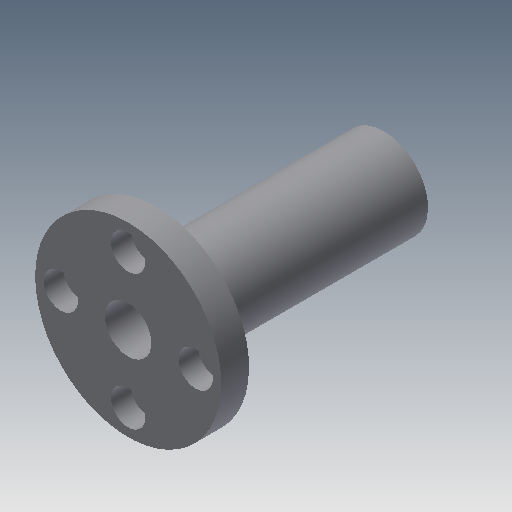
# Autodesk Inventor part: NB_SMF10WW
Saved by Autodesk Inventor 2019.4 (Build 234330000, 330)
## iProperties
Created: 2018-08-09
Part Number: NB_SMF10WW
Material: 一般
Document SubType Name: Modeling
Designer: Owner
Density: 1 g/cm^3
Appearance: 既定
Mass: 16.2699 g
Surface Area: 81.3509 cm^2
Volume: 16.2699 cm^3
Author: Owner
Autodesk Inventor part; units mm, degrees
ref_plane "YZ Plane" through (0, 0, 0) normal (1, 0, 0) x (0, 1, 0)
ref_plane "XZ Plane" through (0, 0, 0) normal (0, 1, 0) x (-1, 0, 0)
ref_plane "XY Plane" through (0, 0, 0) normal (0, 0, 1) x (1, 0, 0)
sketch "スケッチ2" plane through (0, 0, 0) normal (1, 0, 0) x (0, 1, 0)
  line L0 (5, 0) -> (9.5, 0)
  line L1 (9.5, 0) -> (9.5, 49)
  line L2 (9.5, 49) -> (20, 49)
  line L3 (20, 49) -> (20, 55)
  line L4 (20, 55) -> (5, 55)
  line L5 (5, 0) -> (5, 55)
  line L6 (0, -11) -> (0, 66) projected
  point P0 (0, 0)
  point P1 (0, 55)
  dimension "d0" = 9.5
  dimension "d1" = 55
  dimension "d2" = 6
  dimension "d3" = 20
  dimension "d4" = 5
  constraints: 12 end point, 4 perpendicular, 2 point on line, 1 horizontal, 1 vertical, 1 vertical alignment
  measures "d0" distance of point (0, 0) L0.end
  measures "d1" distance between parallel lines of L4 L0
  measures "d2" distance of L2.end L3.end
  measures "d3" distance of L3.end point (0, 55)
  measures "d4" distance from line of point (0, 0) L5
revolve "回転1" add sketch "スケッチ2" angle 360 about axis through (0, 0, -10) along (0, 0, 1)
sketch "スケッチ3" plane through (0, 0, 55) normal (0, 0, 1) x (1, 0, 0)
  circle A0 centre (0, 14.5) radius 3.7
  point P0 (0, 0)
  dimension "d6" = 14.5
  dimension "d7" = 7.4
  constraints: 1 centre point, 1 vertical alignment
  measures "d6" distance of point (0, 0) A0.centre
  measures "d7" diameter of A0
extrude "押し出し1" cut sketch "スケッチ3" against normal blind 4.3
sketch "スケッチ4" plane through (0, 14.5, 50.7) normal (0, 0, 1) x (1, 0, 0)
  circle A0 centre (0, 0) radius 2.2
  circle A1 centre (0, 0) radius 3.7 projected
  point P0 (0, -14.5)
  dimension "d10" = 4.4
  constraints: 1 centre point, 1 concentric
  measures "d10" diameter of A0
extrude "押し出し2" cut sketch "スケッチ4" against normal through all contours A0
pattern_circular "円形状パターン1" count 4 over 360 about axis through (0, 0, -10) along (0, 0, 1) of "押し出し1", "押し出し2"
equation "\"d0\" = 0.5 * D"
equation "\"d1\" = L"
equation "\"d2\" = t"
equation "\"d3\" = 0.5 * Df"
equation "\"d4\" = 0.5 * dr"
equation "\"d6\" = 0.5 * PCD"
equation "\"D\" = 19"
equation "\"L\" = 55"
equation "\"t\" = 6"
equation "\"PCD\" = 29"
equation "\"Df\" = 40"
equation "\"dr\" = 10"
